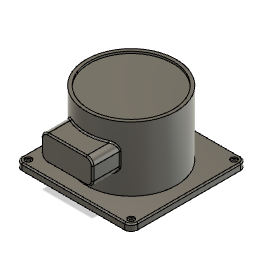
Base (Autodesk Fusion 360 design; units mm, degrees)
Autodesk Fusion 360 part; units mm, degrees
sketch "Sketch1" plane through (0, 0, 0) normal (0, 1, 0) x (1, 0, 0)
  line L0 (90, -90) -> (-90, -90)
  line L1 (-90, -90) -> (-90, 90)
  line L2 (-90, 90) -> (90, 90)
  line L3 (90, 90) -> (90, -90)
  line L4 (90, -90) -> (-90, 90) construction
  line L5 (-90, -90) -> (90, 90) construction
  dimension "d1" = 180
  dimension "d2" = 180
  constraint horizontal L0
  constraint perpendicular L0 L1
  constraint parallel L0 L2
  constraint parallel L1 L3
  constraint coincident L4 origin
  constraint coincident L5 origin
  measures "d1" distance of L1.end L2.end
  measures "d2" distance of L0.end L1.end
extrude "Extrude1" add sketch "Sketch1" along normal blind 10
sketch "Sketch2" plane through (0, 10, 0) normal (0, 1, 0) x (-1, 0, 0)
  line L0 (-90, -90) -> (90, -90)
  line L1 (90, -90) -> (90, 90)
  line L2 (90, 90) -> (-90, 90)
  line L3 (-90, 90) -> (-90, -90)
  circle A0 centre (0, 0) radius 70
  dimension "d5" = 140
  constraint coincident A0.centre origin
  measures "d5" diameter of A0
extrude "Extrude2" add sketch "Sketch2" along normal blind 100 contours A0
sketch "Sketch3" plane through (0, 0, 0) normal (0, 0, 1) x (1, 0, 0)
  line L0 (40, 40) -> (-40, 40)
  line L1 (-40, 40) -> (-40, 80)
  line L2 (-40, 80) -> (40, 80)
  line L3 (40, 80) -> (40, 40)
  line L4 (40, 40) -> (-40, 80) construction
  line L5 (-40, 40) -> (40, 80) construction
  point P0 (0, 60)
  dimension "d8" = 80
  dimension "d9" = 40
  dimension "d10" = 60
  constraint horizontal L0
  constraint perpendicular L0 L1
  constraint parallel L0 L2
  constraint parallel L1 L3
  constraint coincident L4 P0
  constraint coincident L5 P0
  measures "d8" distance of L1.end L2.end
  measures "d9" distance of L0.end L1.end
  measures "d10" distance of origin P0
extrude "Extrude3" add sketch "Sketch3" along normal blind 100
sketch "Sketch4" plane through (0, 110, 0) normal (0, 1, 0) x (-1, 0, 0)
  circle A0 centre (0, 0) radius 70
  circle A1 centre (0, 0) radius 65
  dimension "d13" = -5
extrude "Extrude4" cut sketch "Sketch4" against normal blind 3 contours A1
sketch "Sketch5" plane through (0, 10, 0) normal (0, 1, 0) x (-1, 0, 0)
  circle A0 centre (0, 0) radius 70
  line L0 (-90, -90) -> (90, -90)
  line L1 (90, -90) -> (90, 90)
  line L2 (90, 90) -> (-90, 90)
  line L3 (-90, 90) -> (-90, -90)
  point P0 (80, -80)
  point P1 (-80, -80)
  point P2 (-80, 80)
  point P3 (80, 80)
  dimension "d16" = 10
  dimension "d17" = 10
  dimension "d18" = 10
  dimension "d19" = 10
  dimension "d20" = 10
  dimension "d21" = 10
  dimension "d22" = 10
  dimension "d23" = 10
  measures "d16" distance of L2 P3
  measures "d17" distance of L1 P3
  measures "d18" distance of L3 P2
  measures "d19" distance of L2 P2
  measures "d20" distance of L0 P1
  measures "d21" distance of L3 P1
  measures "d22" distance of L0 P0
  measures "d23" distance of L1 P0
hole "Hole1" at (-80, 10, 80) at (80, 10, 80) at (80, 10, -80) at (-80, 10, -80) direction (0, -1, 0) diameter 5 depth 10 tip angle 118 counterbore diameter 10 counterbore depth 2
fillet "Fillet1" radius 10 8 edges at (-90, 5, 90) (90, 5, 90) (90, 5, -90) (-90, 5, -90) (-40, 80, 78.7228) (-40, 40, 78.7228) (40, 80, 78.7228) (40, 40, 78.7228)
fillet "Fillet2" radius 2 24 edges at (87.0711, 10, -87.0711) (0, 10, -90) (-87.0711, 10, -87.0711) (-90, 10, 0) (-87.0711, 10, 87.0711) (0, 10, 90) (87.0711, 10, 87.0711) (90, 10, 0) (36.9012, 77.2363, 59.4835) (40, 60, 57.4456) (36.9012, 42.7637, 59.4835) (0, 40, 70) (-36.9012, 42.7637, 59.4835) (-40, 60, 57.4456) (-36.9012, 77.2363, 59.4835) (0, 80, 70) (-37.0711, 77.0711, 100) (-40, 60, 100) (-37.0711, 42.9289, 100) (0, 40, 100) (37.0711, 42.9289, 100) (40, 60, 100) (37.0711, 77.0711, 100) (0, 80, 100)
